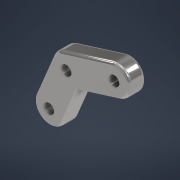
# Autodesk Inventor part: SteelPost
Saved by Autodesk Inventor 2021 (Build 250183000, 183)
## iProperties
Created: 2021-01-30
Part Number: SteelPost
Material: Generic
Document SubType Name: Modeling
Designer: argon
Density: 1 g/cm^3
Appearance: Steel - Polished
Author: argon
Autodesk Inventor part; units mm, degrees
ref_plane "YZ Plane" through (0, 0, 0) normal (1, 0, 0) x (0, 1, 0)
ref_plane "XZ Plane" through (0, 0, 0) normal (0, 1, 0) x (-1, 0, 0)
ref_plane "XY Plane" through (0, 0, 0) normal (0, 0, 1) x (1, 0, 0)
sketch "Sketch1" plane through (0, 0, 0) normal (0, 0, 1) x (1, 0, 0)
  circle A0 centre (2.1561, 2.8874) radius 18
  circle A1 centre (80.1561, 70.6294) radius 18
  circle A2 centre (22.8814, 52.7519) radius 18
  line L0 (74.7929, 87.8119) -> (17.5182, 69.9343)
  line L1 (-14.4653, 9.7959) -> (6.2599, 59.6603)
  line L2 (18.7776, -4.021) -> (39.5029, 45.8434)
  line L3 (85.5194, 53.447) -> (28.2447, 35.5695)
  circle A3 centre (2.1561, 2.8874) radius 6
  circle A4 centre (22.8814, 52.7519) radius 6
  circle A5 centre (80.1561, 70.6294) radius 6
  point P0 (0, 0)
  point P1 (36.2744, 38.0758)
  dimension "d0" = 36
  dimension "d1" = 36
  dimension "d2" = 54
  dimension "d3" = 60
  dimension "d6" = 12
  constraints: 8 end point, 8 point on circle, 8 tangent, 6 centre point, 3 coincident, 3 equal radius
  measures "d0" diameter of A0
  measures "d1" diameter of A1
  measures "d2" distance of A2.centre A0.centre
  measures "d3" distance of A2.centre A1.centre
  measures "d6" diameter of A4
extrude "Extrusion1" add sketch "Sketch1" along normal blind 20
fillet "Fillet1" radius 4 14 edges at (10.748, 66.0477, 20) (-4.1027, 34.7281, 20) (-4.7523, -13.734, 20) (27.526, 17.0274, 20) (97.3386, 75.9927, 20) (60.8969, 45.7614, 20) (46.1555, 78.8731, 20) (10.748, 66.0477, 0) (-4.1027, 34.7281, 0) (-4.7523, -13.734, 0) (27.526, 17.0274, 0) (97.3386, 75.9927, 0) (60.8969, 45.7614, 0) (46.1555, 78.8731, 0)
body "Solid1"
